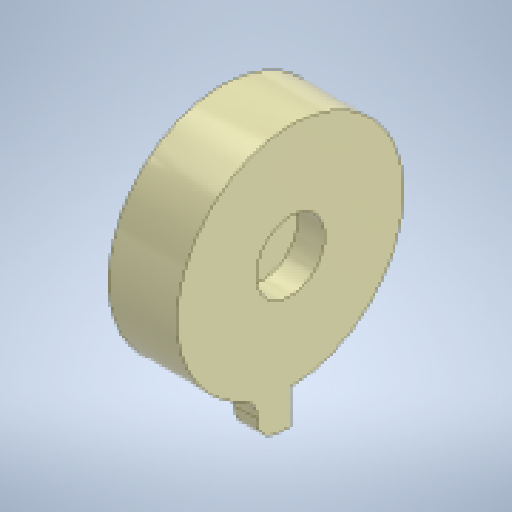
# Autodesk Inventor part: MagToolChanger_Lockplate
Saved by Autodesk Inventor 2023.2 (Build 272271000, 271)
## iProperties
Created: 2022-06-20
Part Number: MagToolChanger_Lockplate
Material: Polycarbonate, Smoke
Document SubType Name: Modeling
Designer: Remo
Density: 1.2 g/cm^3
Appearance: Smooth - Ash
Author: Remo
Autodesk Inventor part; units mm, degrees
ref_plane "YZ Plane" through (0, 0, 0) normal (1, 0, 0) x (0, 1, 0)
ref_plane "XZ Plane" through (0, 0, 0) normal (0, 1, 0) x (-1, 0, 0)
ref_plane "XY Plane" through (0, 0, 0) normal (0, 0, 1) x (1, 0, 0)
sketch "Sketch1" plane through (0, 0, 0) normal (1, 0, 0) x (0, 1, 0)
  circle A0 centre (0, 0) radius 16.4
  circle A1 centre (8.920062, 5.15) radius 5.15
  circle A2 centre (0, 10.3) radius 5.15
  circle A3 centre (-8.920062, 5.15) radius 5.15
  circle A4 centre (-8.920062, -5.15) radius 5.15
  circle A5 centre (0, -10.3) radius 5.15
  circle A6 centre (8.920062, -5.15) radius 5.15
  circle A7 centre (0, 0) radius 2.75
  line L0 (2.2, 1.65) -> (-2.2, 1.65)
  line L1 (-2.2, -1.65) -> (2.2, -1.65)
  point P0 (4.460031, -7.725)
  point P1 (-4.460031, -7.725)
  point P2 (-8.920062, 0)
  point P3 (-4.460031, 7.725)
  point P4 (4.460031, 7.725)
  point P5 (8.920062, 0)
  dimension "d0" = 32.8
  dimension "d1" = 10.3
  dimension "d4" = 360
  dimension "d6" = 5.5
  dimension "d7" = 3.3
  constraints: 8 centre point, 4 end point, 4 point on circle, 2 coincident, 2 parallel, 1 equal radius, 1 horizontal, 1 vertical alignment, 13 other
  measures "d0" diameter of A0
  measures "d1" diameter of A1
  measures "d6" diameter of A7
  measures "d7" distance between parallel lines of L1 L0
extrude "Extrusion1" add sketch "Sketch1" along normal blind 1.6 contours A0 | A1 A6 A5 A4 A3 A2 | L0 A7 | A7 L1
sketch "Sketch2" plane through (1.6, 0, 0) normal (1, 0, 0) x (0, 0, -1)
  circle A0 centre (0, 0) radius 16.4
  arc A1 (7.725, 4.460031) -> (0, 8.920062) centre (5.15, 8.920062) ccw
  arc A2 (7.725, -4.460031) -> (7.725, 4.460031) centre (10.3, 0) ccw
  arc A3 (0, -8.920062) -> (7.725, -4.460031) centre (5.15, -8.920062) ccw
  arc A4 (-7.725, -4.460031) -> (0, -8.920062) centre (-5.15, -8.920062) ccw
  arc A5 (-7.725, 4.460031) -> (-7.725, -4.460031) centre (-10.3, 0) ccw
  arc A6 (0, 8.920062) -> (-7.725, 4.460031) centre (-5.15, 8.920062) ccw
  arc A7 (-7.725, 4.460031) -> (0, 8.920062) centre (-5.15, 8.920062) ccw
  arc A8 (-7.725, -4.460031) -> (-7.725, 4.460031) centre (-10.3, 0) ccw
  arc A9 (0, -8.920062) -> (-7.725, -4.460031) centre (-5.15, -8.920062) ccw
  arc A10 (7.725, -4.460031) -> (0, -8.920062) centre (5.15, -8.920062) ccw
  arc A11 (7.725, 4.460031) -> (7.725, -4.460031) centre (10.3, 0) ccw
  arc A12 (0, 8.920062) -> (7.725, 4.460031) centre (5.15, 8.920062) ccw
  arc A13 (1.65, 2.2) -> (-1.65, 2.2) centre (0, 0) ccw
  line L0 (1.65, 2.2) -> (1.65, -2.2)
  arc A14 (-1.65, -2.2) -> (1.65, -2.2) centre (0, 0) ccw
  line L1 (-1.65, -2.2) -> (-1.65, 2.2)
extrude "Extrusion2" add sketch "Sketch2" along normal blind 4.4 contours A0 | A12 A1 | A2 A11 | A11 A10 A9 A8 A7 A12 | A7 A6 | A3 A10 | A8 A5 | A4 A9
sketch "Sketch3" plane through (6, 0, 0) normal (1, 0, 0) x (0, 0, -1)
  circle A0 centre (0, 0) radius 16.4 projected
  line L0 (-1.65, -2.2) -> (-1.65, 2.2) projected
  arc A1 (1.65, 2.2) -> (-1.65, 2.2) centre (0, 0) ccw projected
  line L1 (1.65, 2.2) -> (1.65, -2.2) projected
  arc A2 (-1.65, -2.2) -> (1.65, -2.2) centre (0, 0) ccw projected
  circle A3 centre (0, 0) radius 5
  dimension "d12" = 10
  constraints: 1 centre point, 1 coincident
  measures "d12" diameter of A3
extrude "Extrusion3" add sketch "Sketch3" along normal blind 4 contours A0
sketch "Sketch4" plane through (10, 0, 0) normal (1, 0, 0) x (0, 0, -1)
  circle A0 centre (0, 0) radius 16.4
  line L0 (0.02309, -16.749984) -> (0.033084, -23.999977)
  line L1 (0.022607, -16.399984) -> (0.02309, -16.749984)
  circle A1 centre (0, 0) radius 21.4
  line L2 (-5.510228, -20.678428) -> (-4.222791, -15.84702)
  point P0 (0.0295, -21.39998)
  dimension "d15" = 5
  dimension "d16" = 15
  constraints: 4 end point, 2 point on circle, 1 coincident, 1 collinear, 1 line through centre, 3 other
  measures "d16" angle of L0 L2
extrude "Extrusion4" add sketch "Sketch4" against normal blind 3.2 contours A0 L1 L0 A1 L2 picked at (-2.782774, -19.518621)
fillet "Fillet1" radius 3 2 edges at (8.4, -15.847, 4.2228) (8.4, -20.6784, 5.5102)
sketch "Sketch5" plane through (6, 0, 0) normal (1, 0, 0) x (0, 0, -1)
  line L0 (-1.65, -2.2) -> (-1.65, 2.2) projected
  arc A0 (-1.65, -2.2) -> (1.65, -2.2) centre (0, 0) ccw projected
  arc A1 (1.65, 2.2) -> (-1.65, 2.2) centre (0, 0) ccw projected
  line L1 (1.65, 2.2) -> (1.65, -2.2) projected
extrude "Extrusion5" add sketch "Sketch5" against normal blind 0.2
sketch "Sketch6" plane through (0, 0, 0) normal (-1, 0, 0) x (0, 0, 1)
  circle A0 centre (0, 0) radius 16.4
  arc A1 (0, 8.920062) -> (-7.725, 4.460031) centre (-5.15, 8.920062) ccw
  arc A2 (7.725, 4.460031) -> (0, 8.920062) centre (5.15, 8.920062) ccw
  arc A3 (7.725, -4.460031) -> (7.725, 4.460031) centre (10.3, 0) ccw
  arc A4 (0, -8.920062) -> (7.725, -4.460031) centre (5.15, -8.920062) ccw
  arc A5 (-7.725, -4.460031) -> (0, -8.920062) centre (-5.15, -8.920062) ccw
  arc A6 (-7.725, 4.460031) -> (-7.725, -4.460031) centre (-10.3, 0) ccw
  arc A7 (0, 8.920062) -> (7.725, 4.460031) centre (5.15, 8.920062) ccw
  arc A8 (-7.725, 4.460031) -> (0, 8.920062) centre (-5.15, 8.920062) ccw
  arc A9 (-7.725, -4.460031) -> (-7.725, 4.460031) centre (-10.3, 0) ccw
  arc A10 (0, -8.920062) -> (-7.725, -4.460031) centre (-5.15, -8.920062) ccw
  arc A11 (7.725, -4.460031) -> (0, -8.920062) centre (5.15, -8.920062) ccw
  arc A12 (7.725, 4.460031) -> (7.725, -4.460031) centre (10.3, 0) ccw
  arc A13 (1.65, 2.2) -> (-1.65, 2.2) centre (0, 0) ccw
  line L0 (1.65, -2.2) -> (1.65, 2.2)
  arc A14 (-1.65, -2.2) -> (1.65, -2.2) centre (0, 0) ccw
  line L1 (-1.65, 2.2) -> (-1.65, -2.2)
  circle A15 centre (0, 0) radius 8.920062 construction
  circle A16 centre (0, 0) radius 9.920062
  circle A17 centre (0, 0) radius 7.920062
  point P0 (6.809378, -4.044719)
  point P1 (0.098141, -7.919454)
  point P2 (0.097925, -9.919578)
  point P3 (8.541645, -5.044594)
  point P4 (-0.098141, -7.919454)
  point P5 (-6.809378, -4.044719)
  point P6 (-7.725, -4.460031)
  point P7 (-7.725, -4.460031)
  point P8 (-7.725, -4.460031)
  point P9 (-7.725, -4.460031)
  point P10 (-8.541645, -5.044594)
  point P11 (-0.097925, -9.919578)
  point P12 (-6.907518, -3.874735)
  point P13 (-6.907518, 3.874735)
  point P14 (-8.639569, 4.874984)
  point P15 (-8.639569, -4.874984)
  point P16 (6.907518, -3.874735)
  point P17 (8.639569, -4.874984)
  point P18 (8.639569, 4.874984)
  point P19 (6.907518, 3.874735)
  point P20 (0.098141, 7.919454)
  point P21 (6.809378, 4.044719)
  point P22 (8.541645, 5.044594)
  point P23 (0.097925, 9.919578)
  point P24 (0, 8.920062)
  point P25 (0, 8.920062)
  point P26 (0, 8.920062)
  point P27 (0, 8.920062)
  point P28 (-6.809378, 4.044719)
  point P29 (-0.098141, 7.919454)
  point P30 (-0.097925, 9.919578)
  point P31 (-8.541645, 5.044594)
  dimension "d25" = 1
  dimension "d26" = 1
  constraints: 3 coincident, 2 centre point, 3 other
extrude "Extrusion6" cut sketch "Sketch6" against normal up to surface (1.6 mm away) contours A8 A17 A1 A16 | A1 A16 A2 | A2 A16 A7 A17 | A7 A17 A8 | A1 A6 A16 | A16 A3 A2 | A7 A12 A17 | A17 A9 A8 | A9 A17 A6 A16 | A3 A16 A12 A17 | A6 A5 A16 | A16 A4 A3 | A12 A11 A17 | A17 A10 A9 | A10 A17 A5 A16 | A4 A16 A11 A17 | A5 A4 A16 | A11 A10 A17
fillet "Fillet2" radius 0.4 24 edges at (0.8, 7.9195, -0.0981) (0.8, 7.9195, 0.0981) (0.8, 9.9196, 0.0979) (0.8, 9.9196, -0.0979) (0.8, 4.875, -8.6396) (0.8, 5.0446, -8.5416) (0.8, 4.0447, -6.8094) (0.8, 3.8747, -6.9075) (0.8, -5.0446, -8.5416) (0.8, -4.875, -8.6396) (0.8, -9.9196, 0.0979) (0.8, -9.9196, -0.0979) (0.8, -5.0446, 8.5416) (0.8, -4.875, 8.6396) (0.8, -4.0447, 6.8094) (0.8, -3.8747, 6.9075) (0.8, 3.8747, 6.9075) (0.8, 4.0447, 6.8094) (0.8, -4.0447, -6.8094) (0.8, -3.8747, -6.9075) (0.8, -7.9195, -0.0981) (0.8, -7.9195, 0.0981) (0.8, 5.0446, 8.5416) (0.8, 4.875, 8.6396)
equation "\"d26\" = d25"
body "Solid1"
